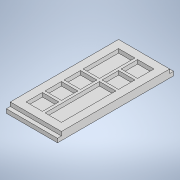
# Autodesk Inventor part: Лого ШП
Saved by Autodesk Inventor 2020 (Build 240168000, 168)
## iProperties
Created: 2021-06-18
Part Number: Лого ШП
Material: Типовые
Document SubType Name: Modeling
Designer: Антон
Density: 1 g/cm^3
Appearance: По умолчанию
Author: Антон
Autodesk Inventor part; units mm, degrees
ref_plane "YZ Plane" through (0, 0, 0) normal (1, 0, 0) x (0, 1, 0)
ref_plane "XZ Plane" through (0, 0, 0) normal (0, 1, 0) x (-1, 0, 0)
ref_plane "XY Plane" through (0, 0, 0) normal (0, 0, 1) x (1, 0, 0)
sketch "Эскиз1" plane through (0, 0, 0) normal (0, 1, 0) x (-1, 0, 0)
  line L0 (0, 0) -> (13, 0)
  line L1 (13, 0) -> (13, -27.5)
  line L2 (13, -27.5) -> (0, -27.5)
  line L3 (0, -27.5) -> (0, 0)
  line L4 (11, -2) -> (6.8333, -2)
  line L5 (6.8333, -2) -> (6.8333, -6.1667)
  line L6 (6.8333, -6.1667) -> (11, -6.1667)
  line L7 (11, -6.1667) -> (11, -2)
  line L8 (11, -6.8333) -> (6.8333, -6.8333)
  line L9 (6.8333, -6.8333) -> (6.8333, -11)
  line L10 (6.8333, -11) -> (11, -11)
  line L11 (11, -11) -> (11, -6.8333)
  line L12 (11, -11.6667) -> (6.8333, -11.6667)
  line L13 (6.8333, -11.6667) -> (6.8333, -15.8333)
  line L14 (6.8333, -15.8333) -> (11, -15.8333)
  line L15 (11, -15.8333) -> (11, -11.6667)
  line L16 (11, -16.5) -> (6.8333, -16.5)
  line L17 (6.8333, -16.5) -> (6.8333, -25.5)
  line L18 (6.8333, -25.5) -> (11, -25.5)
  line L19 (11, -25.5) -> (11, -16.5)
  line L20 (6.1667, -16.5) -> (2, -16.5)
  line L21 (2, -16.5) -> (2, -20.6667)
  line L22 (2, -20.6667) -> (6.1667, -20.6667)
  line L23 (6.1667, -20.6667) -> (6.1667, -16.5)
  line L24 (6.1667, -21.3333) -> (2, -21.3333)
  line L25 (2, -21.3333) -> (2, -25.5)
  line L26 (2, -25.5) -> (6.1667, -25.5)
  line L27 (6.1667, -25.5) -> (6.1667, -21.3333)
  line L28 (6.1667, -2) -> (2, -2)
  line L29 (2, -2) -> (2, -15.8333)
  line L30 (2, -15.8333) -> (6.1667, -15.8333)
  line L31 (6.1667, -15.8333) -> (6.1667, -2)
  line L32 (8.9167, -6.1667) -> (8.9167, -6.8333)
  line L33 (8.9167, -11) -> (8.9167, -11.6667)
  line L34 (8.9167, -15.8333) -> (8.9167, -16.5)
  line L35 (4.0833, -15.8333) -> (4.0833, -16.5)
  line L36 (4.0833, -20.6667) -> (4.0833, -21.3333)
  line L37 (8.9167, -2) -> (8.9167, 0)
  line L38 (8.9167, -25.5) -> (8.9167, -27.5)
  line L39 (11, -8.9167) -> (13, -8.9167)
  line L40 (2, -8.9167) -> (0, -8.9167)
  line L41 (6.8333, -8.9167) -> (6.1667, -8.9167)
  dimension "d0" = 13
  dimension "d1" = 27.5
  dimension "d9" = 2
  constraints: 84 end point, 18 equal length, 16 midpoint, 16 parallel, 11 perpendicular, 9 collinear, 8 horizontal, 4 point on line, 1 vertical
  measures "d0" distance of L1.end L2.end
  measures "d1" distance of L0.end L1.end
  measures "d9" distance of L39.start L39.end
extrude "Выдавливание1" add sketch "Эскиз1" along normal blind 1 contours L0 L37 L4 L5 L6 L32 L8 L9 L41 L31 L28 L29 L40 L3 | L0 L1 L39 L11 L8 L32 L6 L7 L4 L37 | L40 L29 L30 L31 L41 L9 L10 L33 L12 L13 L14 L34 L16 L17 L18 L38 L2 L3 | L1 L2 L38 L18 L19 L16 L34 L14 L15 L12 L33 L10 L11 L39
sketch "Эскиз2" plane through (0, 0, 0) normal (0, -1, 0) x (1, 0, 0)
  line L0 (0, 0) -> (0, -27.5) projected
  line L1 (-13, 0) -> (0, 0) projected
  line L2 (-13, -27.5) -> (-13, 0) projected
  line L3 (0, -27.5) -> (-13, -27.5) projected
  line L4 (-6.1667, -15.8333) -> (-2, -15.8333) projected
  line L5 (-6.1667, -2) -> (-6.1667, -15.8333) projected
  line L6 (-2, -2) -> (-6.1667, -2) projected
  line L7 (-2, -15.8333) -> (-2, -2) projected
  line L8 (-2, -25.5) -> (-2, -21.3333) projected
  line L9 (-6.1667, -25.5) -> (-2, -25.5) projected
  line L10 (-6.1667, -21.3333) -> (-6.1667, -25.5) projected
  line L11 (-2, -21.3333) -> (-6.1667, -21.3333) projected
  line L12 (-6.8333, -11.6667) -> (-11, -11.6667) projected
  line L13 (-6.8333, -15.8333) -> (-6.8333, -11.6667) projected
  line L14 (-11, -15.8333) -> (-6.8333, -15.8333) projected
  line L15 (-11, -11.6667) -> (-11, -15.8333) projected
  line L16 (-11, -16.5) -> (-11, -25.5) projected
  line L17 (-6.8333, -16.5) -> (-11, -16.5) projected
  line L18 (-6.8333, -25.5) -> (-6.8333, -16.5) projected
  line L19 (-11, -25.5) -> (-6.8333, -25.5) projected
  line L20 (-11, -11) -> (-6.8333, -11) projected
  line L21 (-11, -6.8333) -> (-11, -11) projected
  line L22 (-6.8333, -6.8333) -> (-11, -6.8333) projected
  line L23 (-6.8333, -11) -> (-6.8333, -6.8333) projected
  line L24 (-11, -2) -> (-11, -6.1667) projected
  line L25 (-6.8333, -2) -> (-11, -2) projected
  line L26 (-6.8333, -6.1667) -> (-6.8333, -2) projected
  line L27 (-11, -6.1667) -> (-6.8333, -6.1667) projected
  line L28 (-2, -20.6667) -> (-2, -16.5) projected
  line L29 (-6.1667, -20.6667) -> (-2, -20.6667) projected
  line L30 (-6.1667, -16.5) -> (-6.1667, -20.6667) projected
  line L31 (-2, -16.5) -> (-6.1667, -16.5) projected
extrude "Выдавливание2" add sketch "Эскиз2" along normal blind 1 contours L0 L3 L2 L1 | L5 L6 L7 L4 | L9 L10 L11 L8 | L13 L14 L15 L12 | L17 L18 L19 L16 | L21 L22 L23 L20 | L25 L26 L27 L24 | L29 L30 L31 L28
sketch "Эскиз3" plane through (-13, 1, 0) normal (0, 0, 1) x (1, 0, 0)
  line L0 (0, -2) -> (13, -2)
  line L1 (13, -2) -> (13, -1)
  line L2 (13, -1) -> (0, -1)
  line L3 (0, -1) -> (0, -2)
  line L4 (13, -2) -> (13, 0) projected
  line L5 (0, -2) -> (0, 0) projected
  line L6 (13, -2) -> (0, -2) projected
  dimension "d14" = 1
  constraints: 8 end point, 3 collinear, 2 parallel, 1 horizontal, 1 perpendicular
  measures "d14" distance of L0.end L1.end
extrude "Выдавливание3" add sketch "Эскиз3" along normal blind 1
sketch "Эскиз4" plane through (0, 1, -27.5) normal (0, 0, -1) x (-1, 0, 0)
  line L0 (6.8333, -1) -> (11, -1) projected
  line L1 (13, -2) -> (0, -2) projected
  line L2 (0, -2) -> (0, -1) projected
  line L3 (0, -1) -> (13, -1) projected
  line L4 (13, -1) -> (13, -2) projected
extrude "Выдавливание4" add sketch "Эскиз4" along normal blind 1
